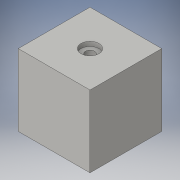
# Autodesk Inventor part: Part1
Saved by Autodesk Inventor 2016 SP2 (Build 200236200, 236)
## iProperties
Created: 2017-01-05
Part Number: Part1
Material: Generic
Document SubType Name: Modeling
Designer: amarrufo01
Density: 1 g/cm^3
Appearance: Default
Author: amarrufo01
Autodesk Inventor part; units mm, degrees
ref_plane "YZ Plane" through (0, 0, 0) normal (1, 0, 0) x (0, 1, 0)
ref_plane "XZ Plane" through (0, 0, 0) normal (0, 1, 0) x (-1, 0, 0)
ref_plane "XY Plane" through (0, 0, 0) normal (0, 0, 1) x (1, 0, 0)
sketch "Sketch1" plane through (0, 0, 0) normal (0, 1, 0) x (-1, 0, 0)
  line L0 (-3.9786, 20.196) -> (97.6214, 20.196)
  line L1 (97.6214, 20.196) -> (97.6214, -81.404)
  line L2 (97.6214, -81.404) -> (-3.9786, -81.404)
  line L3 (-3.9786, -81.404) -> (-3.9786, 20.196)
  point P0 (0, 0)
  dimension "d0" = 101.6
  dimension "d1" = 101.6
  constraints: 8 end point, 2 parallel, 1 horizontal, 1 perpendicular
  measures "d0" distance of L1.end L2.end
  measures "d1" distance of L0.end L1.end
extrude "Extrusion1" add sketch "Sketch1" along normal blind 101.6
sketch "Sketch2" plane through (0, 101.6, 0) normal (0, 1, 0) x (1, 0, 0)
  line L0 (3.9786, 81.404) -> (-97.6214, 81.404) projected
  line L1 (-97.6214, -20.196) -> (3.9786, -20.196) projected
  circle A0 centre (-46.8214, 30.604) radius 25.4
  point P0 (0, 0)
  dimension "d4" = 50.8
  constraints: 1 centre point
  measures "d4" diameter of A0
hole "Hole1" at (-46.8214, 101.6, -30.604) direction (0, -1, 0) diameter 12.7 depth 76.2 tip angle 118 counterbore diameter 25.4 counterbore depth 6.35
body "Solid1"
